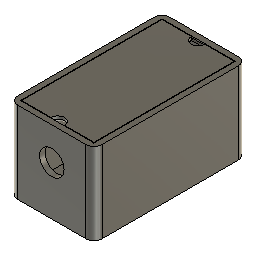
bicycle_dynamo_charger (Autodesk Fusion 360 design; units mm, degrees)
part number: 2026-06-18-18-18-58-321
Autodesk Fusion 360 part; units mm, degrees
sketch "Sketch1" plane through (0, 0, 0) normal (0, 0, 1) x (1, 0, 0)
  line L0 (0, 0) -> (27, 0)
  line L1 (27, 0) -> (27, 52)
  line L2 (27, 52) -> (0, 52)
  line L3 (0, 52) -> (0, 0)
  line L4 (-2, 54) -> (-2, -2)
  line L5 (-2, -2) -> (29, -2)
  line L6 (29, -2) -> (29, 54)
  line L7 (29, 54) -> (-2, 54)
  circle A0 centre (24, 49) radius 2.2
  circle A1 centre (24, 3) radius 2.2
  line L8 (-2, 26) -> (60, 26) construction
  line L9 (13.5, -2) -> (13.5, 65) construction
  circle A2 centre (3, 49) radius 2.2
  circle A3 centre (3, 3) radius 2.2
  dimension "d1" = 27
  dimension "d2" = 52
  dimension "d3" = 2
  dimension "d4" = 4.4
  dimension "d5" = 4.4
  dimension "d6" = 46
  dimension "d7" = 10.5
  constraint horizontal L0
  constraint vertical L1
  constraint horizontal L2
  constraint vertical L3
  constraint coincident L0.start L3.end
  constraint midpoint L4 L8.start
  constraint perpendicular L6 L8
  constraint symmetric A0.centre A1.centre L8
  constraint midpoint L5 L9.start
  constraint perpendicular L2 L9
  constraint symmetric A0 L9 A2
  constraint symmetric A1 L9 A3
  measures "d1" distance of L0.start L0.end
  measures "d2" distance of L0.start L2.end
  measures "d4" diameter of A0
  measures "d5" diameter of A1
  measures "d6" vertical distance of A0.centre A1.centre
  measures "d7" distance of A0.centre L9
extrude "Extrude1" add sketch "Sketch1" along normal blind 4 contours L0 L1 L2 L3 makes body 1
extrude "Extrude2" add sketch "Sketch1" along normal blind 30 contours L4 L5 L6 L7 bodies 1
sketch "Sketch2" plane through (0, -2, 0) normal (0, -1, 0) x (1, 0, 0)
  line L0 (-2, 0) -> (29, 0)
  line L1 (29, 0) -> (29, 30)
  line L2 (29, 30) -> (-2, 30)
  line L3 (-2, 30) -> (-2, 0)
  circle A0 centre (13.5, 18) radius 4.5
  line L4 (31, 2) -> (-6, 2) construction
  line L5 (-2, 0) -> (60, 0)
  dimension "d12" = 9
  dimension "d13" = 2
  dimension "d14" = 16
  dimension "d15" = 31
  dimension "d16" = 15.5
  constraint perpendicular L3 L4
  measures "d12" diameter of A0
  measures "d13" distance of L4 L5
  measures "d14" distance of A0.centre L4
  measures "d15" distance of L1 L3
  measures "d16" distance of L1 A0.centre
extrude "Extrude3" cut sketch "Sketch2" against normal blind 4 contours A0 bodies 1
sketch "Sketch3" plane through (-2, 0, 0) normal (-1, 0, 0) x (0, -1, 0)
  line L0 (-54, 0) -> (2, 0)
  line L1 (2, 0) -> (2, 30)
  line L2 (2, 30) -> (-54, 30)
  line L3 (-54, 30) -> (-54, 0)
  line L4 (-45.499, 21.9483) -> (-36.499, 21.9483)
  line L5 (-36.499, 16.0517) -> (-45.499, 16.0517)
  line L6 (-33.4991, 21.9483) -> (-48.5009, 16.0517) construction
  line L7 (-48.2991, 21.9483) -> (-33.5476, 16.0517) construction
  line L8 (-54, 0) -> (2, 0)
  arc A0 (-45.499, 21.9483) -> (-48.4985, 19) centre (-45.499, 18.9483) ccw
  arc A1 (-33.4995, 19) -> (-36.499, 21.9483) centre (-36.499, 18.9483) ccw
  arc A2 (-36.499, 16.0517) -> (-33.4995, 19) centre (-36.499, 19.0517) ccw
  arc A3 (-48.4985, 19) -> (-45.499, 16.0517) centre (-45.499, 19.0517) ccw
  point P0 (-41, 19)
  dimension "d19" = 14.8
  dimension "d20" = 5.9
  dimension "d21" = 19
  dimension "d22" = 13
  dimension "d25" = 3
  dimension "d26" = 3
  dimension "d27" = 3
  dimension "d28" = 3
  constraint horizontal L4
  constraint horizontal L5
  constraint midpoint L6 P0
  constraint coincident L7.start L4
  constraint tangent L4 A0
  constraint coincident L6.start L4
  constraint tangent L4 A1
  constraint coincident L7.end L5
  constraint tangent L5 A2
  constraint coincident A1.start A2.end
  constraint coincident L6.end L5
  constraint tangent L5 A3
  constraint coincident A0.end A3.start
  measures "d19" distance of L7.start L6.start
  measures "d20" distance of L7.start L6.end
  measures "d21" distance of P0 L8
  measures "d22" distance of L3 P0
  measures "d25" radius of A0
  measures "d26" radius of A1
  measures "d27" radius of A2
  measures "d28" radius of A3
extrude "Extrude4" cut sketch "Sketch3" against normal blind 4 contours L4 L5 A0 A1 A2 A3 bodies 1
fillet "Fillet2" radius 3 4 edges at (29, -2, 15) (-2, -2, 15) (-2, 54, 15) (29, 54, 15) on bodies 1
sketch "Sketch4" plane through (0, 0, 4) normal (0, 0, 1) x (-1, 0, 0)
  circle A0 centre (-3, -49) radius 2.2
  circle A1 centre (-24, -3) radius 2.2
  circle A2 centre (-3, -3) radius 2.2
  circle A3 centre (-24, -49) radius 2.2
  line L0 (0, -52) -> (0, 0)
  line L1 (0, 0) -> (-27, 0)
  line L2 (-27, 0) -> (-27, -52)
  line L3 (-27, -52) -> (0, -52)
  circle A4 centre (-24, -3) radius 3
  circle A5 centre (-3, -3) radius 3
  circle A6 centre (-24, -49) radius 3
  circle A7 centre (-3, -49) radius 3
  dimension "d33" = 6
  dimension "d34" = 6
  dimension "d35" = 6
  dimension "d36" = 6
  constraint concentric A1 A4
  constraint concentric A2 A5
  constraint concentric A3 A6
  constraint concentric A0 A7
  measures "d33" diameter of A4
  measures "d34" diameter of A5
  measures "d35" diameter of A6
  measures "d36" diameter of A7
extrude "Extrude5" cut sketch "Sketch4" against normal blind 2 contours L0 L1 L2 L3 A4 A5 A6 A7 bodies 1
sketch "Sketch5" plane through (0, 0, 30) normal (0, 0, 1) x (-1, 0, 0)
  arc A0 (-29, -51) -> (-26, -54) centre (-26, -51) ccw
  line L0 (-26, -54) -> (-1, -54)
  arc A1 (-1, -54) -> (2, -51) centre (-1, -51) ccw
  line L1 (2, -51) -> (2, -1)
  arc A2 (2, -1) -> (-1, 2) centre (-1, -1) ccw
  line L2 (-1, 2) -> (-26, 2)
  arc A3 (-26, 2) -> (-29, -1) centre (-26, -1) ccw
  line L3 (-29, -1) -> (-29, -51)
  line L4 (0, 0) -> (0, -52)
  line L5 (0, -52) -> (-27, -52)
  line L6 (-27, -52) -> (-27, 0)
  line L7 (-27, 0) -> (0, 0)
  line L8 (-0.2, -0.2) -> (-0.2, -51.8)
  line L9 (-0.2, -51.8) -> (-26.8, -51.8)
  line L10 (-26.8, -51.8) -> (-26.8, -0.2)
  line L11 (-26.8, -0.2) -> (-0.2, -0.2)
  dimension "d39" = 0.2
extrude "Extrude6" add sketch "Sketch5" against normal blind 2 separate body contours L8 L9 L10 L11 makes body 2
ref_plane "WorkPlane1" through (13.5, 26, 29) normal (0, 0, 1) x (-1, 0, 0)
sketch "Sketch6" plane through (0, 0, 29) normal (0, 0, 1) x (1, 0, 0)
  line L0 (0.2, 0.2) -> (0.2, 51.8)
  line L1 (26.8, 0.2) -> (0.2, 0.2)
  line L2 (26.8, 51.8) -> (26.8, 0.2)
  line L3 (0.2, 51.8) -> (26.8, 51.8)
ref_plane "WorkPlane2" through (0.2, 27.067, 29.1759) normal (0, -1, 0) x (-1, 0, 0)
sketch "Sketch7" plane through (0, 27.067, 0) normal (0, -1, 0) x (-1, 0, 0)
  circle A0 centre (-26.8, -29) radius 0.5
  dimension "d44" = 1
  measures "d44" diameter of A0
sweep "Sweep1" add profiles "Sketch7" path "Sketch6" along L1 L0 L3 L2 section 1 bodies 2
combine "Combine1" operation cut target body 1 tool bodies 2 keep tools
sketch "Sketch8" plane through (0, 0, 30) normal (0, 0, 1) x (-1, 0, 0)
  line L0 (-26.8, -0.2) -> (-26.8, -51.8)
  line L1 (-26.8, -51.8) -> (-0.2, -51.8)
  line L2 (-0.2, -51.8) -> (-0.2, -0.2)
  line L3 (-0.2, -0.2) -> (-26.8, -0.2)
  arc A0 (-16, -0.2) -> (-11, -0.2) centre (-13.5, -0.2) ccw
  arc A1 (-11, -51.8) -> (-16, -51.8) centre (-13.5, -51.8) ccw
  dimension "d51" = 5
  dimension "d52" = 5
  constraint midpoint L1 A1.centre
  constraint midpoint L3 A0.centre
  constraint coincident L3 A0.end
  constraint coincident L3 A0.start
  constraint coincident L1 A1.end
  constraint coincident L1 A1.start
  measures "d51" diameter of A1
  measures "d52" diameter of A0
extrude "Extrude7" cut sketch "Sketch8" against normal blind 3 contours L3 A0 | L1 A1 bodies 2
delete_face "DeleteFace1" 1 faces at (12.6667, 0.2, 29.1667) on bodies 2
delete_face "DeleteFace2" 1 faces at (14.3333, 51.8, 29.1667) on bodies 2
move_face "OffsetFaces1" offset -0.1 6 faces at (27.2966, 17.2434, 29.058) (23.2313, 51.8545, 28.503) (3.7687, 51.8545, 28.503) (-0.2966, 34.7566, 29.058) (3.7687, 0.1455, 28.503) (23.2313, 0.1455, 28.503) on bodies 2
fillet "Fillet3" radius 1 1 faces at (22.6711, 18.1757, 28) on bodies 2
equation "d16 = d15 / 2"
